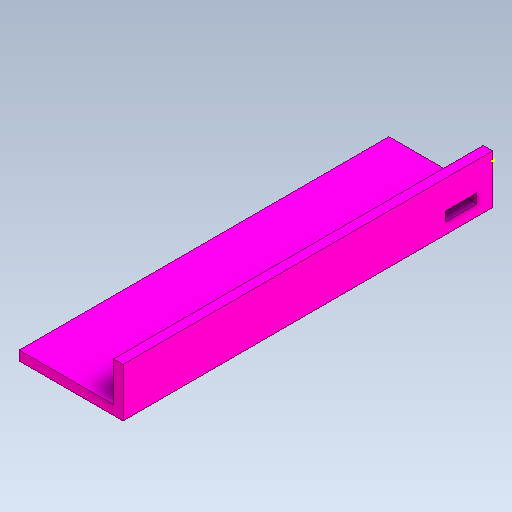
# Autodesk Inventor part: hull_servo_cable_lid
Saved by Autodesk Inventor 2020 (Build 240168000, 168)
## iProperties
Created: 2019-09-19
Part Number: hull_servo_cable_lid
Material: Generic
Document SubType Name: Modeling
Designer: suchanek
Density: 1 g/cm^3
Appearance: Default
Author: suchanek
Autodesk Inventor part; units mm, degrees
ref_plane "YZ Plane" through (0, 0, 0) normal (1, 0, 0) x (0, 1, 0)
sketch "Sketch1" plane through (0, 0, 0) normal (0, 0, 1) x (1, 0, 0)
  line L0 (-39.0826, -45) -> (39.0826, -45) projected
  line L1 (39.0826, -45) -> (36.4496, -25) projected
  line L2 (31.4064, -25) -> (36.4496, -25) projected
  line L3 (28.1151, 0) -> (31.4064, -25) projected
  line L4 (0.5, 0) -> (28.1151, 0) projected
  line L5 (0.5, 2.5) -> (0.5, 0) projected
  line L6 (-2.5, 2.5) -> (0.5, 2.5) projected
  line L7 (-2.5, 0) -> (-2.5, 2.5) projected
  line L8 (-28.1151, 0) -> (-2.5, 0) projected
  line L9 (-29.4316, -10) -> (-28.1151, 0) projected
  line L10 (-32.3266, -10) -> (-29.4316, -10) projected
  line L11 (-32.3266, -13) -> (-32.3266, -10) projected
  line L12 (-29.8266, -13) -> (-32.3266, -13) projected
  line L13 (-31.4064, -25) -> (-29.8266, -13) projected
  line L14 (-36.4496, -25) -> (-31.4064, -25) projected
  line L15 (-36.4496, -25) -> (-39.0826, -45) projected
  line L16 (-32.3266, -10) -> (-2.5, -10)
  line L17 (-2.5, -10) -> (-2.5, -13)
  line L18 (-2.5, -13) -> (-32.3266, -13)
  line L19 (-32.3266, -13) -> (-32.3266, -10)
  line L20 (-2.5, 2.5) -> (0.5, 2.5)
  line L21 (0.5, 2.5) -> (0.5, -13)
  line L22 (0.5, -13) -> (-2.5, -13)
  line L23 (-2.5, -13) -> (-2.5, 2.5)
  point P0 (0, 0)
  point P1 (-2.5, -10)
  constraints: 16 end point, 4 parallel, 2 horizontal, 2 perpendicular, 2 point on line
ref_plane "Work Plane1" through (-36.4496, -25, 120) normal (0, 0, 1) x (1, 0, 0)
ref_plane "Work Plane2" through (-35.4409, -25, 117) normal (0, 0, 1) x (1, 0, 0)
extrude "Extrusion1" add sketch "Sketch1" along normal up to surface (117 mm away) contours L12 L11 L10 L16 L17 L18 | L17 L23 L7 L6 L5 L21 L22
sketch "Sketch2" plane through (0.5, -13, 0) normal (1, 0, 0) x (0, 0, -1)
  point P0 (0, 13)
sketch "Sketch3" plane through (0.5, -13, 0) normal (1, 0, 0) x (0, 0, -1)
  line L0 (-15, 6.5) -> (-5, 6.5)
  line L1 (-5, 6.5) -> (-5, 3.5)
  line L2 (-5, 3.5) -> (-15, 3.5)
  line L3 (-15, 3.5) -> (-15, 6.5)
  line L4 (0, 3) -> (-117, 3) projected
  line L5 (0, 0) -> (0, 15.5) projected
  point P0 (0, 13)
  dimension "d2" = 10
  dimension "d3" = 3
  dimension "d4" = 0.5
  dimension "d5" = 5
  constraints: 8 end point, 2 parallel, 1 horizontal, 1 perpendicular
  measures "d2" distance of L1.end L2.end
  measures "d3" distance of L0.end L1.end
  measures "d4" distance between parallel lines of L2 L4
  measures "d5" distance between parallel lines of L5 L1
extrude "Extrusion2" cut sketch "Sketch3" against normal through all
body "Solid1"
